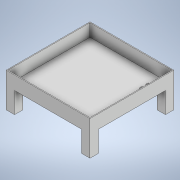
# Autodesk Inventor part: grow bed
Saved by Autodesk Inventor 2020 (Build 240168000, 168)
## iProperties
Created: 2019-09-26
Part Number: grow bed
Material: Generic
Document SubType Name: Modeling
Designer: Abbas
Density: 1 g/cm^3
Appearance: Default
Author: Abbas
Autodesk Inventor part; units mm, degrees
ref_plane "YZ Plane" through (0, 0, 0) normal (1, 0, 0) x (0, 1, 0)
ref_plane "XZ Plane" through (0, 0, 0) normal (0, 1, 0) x (-1, 0, 0)
ref_plane "XY Plane" through (0, 0, 0) normal (0, 0, 1) x (1, 0, 0)
sketch "Sketch2" plane through (0, 0, 0) normal (0, 1, 0) x (-1, 0, 0)
  line L0 (7.9621, 7.1123) -> (-1992.0379, 7.1123)
  line L1 (-1992.0379, 7.1123) -> (-1992.0379, -1992.8877)
  line L2 (-1992.0379, -1992.8877) -> (7.9621, -1992.8877)
  line L3 (7.9621, -1992.8877) -> (7.9621, 7.1123)
  point P0 (0, 0)
  dimension "d0" = 2000
  dimension "d1" = 2000
  constraints: 8 end point, 2 parallel, 1 horizontal, 1 perpendicular
  measures "d0" distance of L2.end L1.end
  measures "d1" distance of L1.end L0.end
extrude "Extrusion1" add sketch "Sketch2" along normal blind 320
sketch "Sketch5" plane through (0, 320, 0) normal (0, 1, 0) x (1, 0, 0)
  line L0 (12.0379, 12.8877) -> (1972.0379, 12.8877)
  line L1 (1972.0379, 12.8877) -> (1972.0379, 1972.8877)
  line L2 (1972.0379, 1972.8877) -> (12.0379, 1972.8877)
  line L3 (12.0379, 1972.8877) -> (12.0379, 12.8877)
  line L4 (-7.9621, -7.1123) -> (1992.0379, -7.1123) projected
  line L5 (1992.0379, -7.1123) -> (1992.0379, 1992.8877) projected
  dimension "d7" = 1960
  dimension "d8" = 20
  dimension "d9" = 1960
  dimension "d10" = 20
  constraints: 8 end point, 2 parallel, 1 horizontal, 1 perpendicular
  measures "d7" distance of L0.end L1.end
  measures "d8" distance between parallel lines of L4 L0
  measures "d9" distance of L1.end L2.end
  measures "d10" distance between parallel lines of L5 L1
extrude "Extrusion2" cut sketch "Sketch5" against normal blind 300
sketch "Sketch6" plane through (0, 20, 0) normal (0, 1, 0) x (1, 0, 0)
  circle A0 centre (1692.0379, 1692.8877) radius 50
  circle A1 centre (1692.0379, 1542.8877) radius 50
  line L0 (1992.0379, 1992.8877) -> (-7.9621, 1992.8877) projected
  line L1 (1992.0379, -7.1123) -> (1992.0379, 1992.8877) projected
  point P0 (0, 0)
  dimension "d13" = 100
  dimension "d14" = 100
  dimension "d15" = 300
  dimension "d16" = 300
  dimension "d17" = 300
  dimension "d18" = 150
  constraints: 2 centre point
  measures "d13" diameter of A1
  measures "d14" diameter of A0
  measures "d15" distance from line of L0 A0.centre
  measures "d16" distance from line of L1 A0.centre
  measures "d17" distance from line of L1 A1.centre
  measures "d18" distance of A1.centre A0.centre
extrude "Extrusion3" cut sketch "Sketch6" against normal blind 300
sketch "Sketch7" plane through (0, 0, 0) normal (0, -1, 0) x (1, 0, 0)
  line L0 (1992.0379, 7.1123) -> (1792.0379, 7.1123)
  line L1 (1792.0379, 7.1123) -> (1792.0379, -192.8877)
  line L2 (1792.0379, -192.8877) -> (1992.0379, -192.8877)
  line L3 (1992.0379, -192.8877) -> (1992.0379, 7.1123)
  line L4 (-7.9621, 7.1123) -> (1992.0379, 7.1123) projected
  line L5 (-7.9621, 7.1123) -> (192.0379, 7.1123)
  line L6 (192.0379, 7.1123) -> (192.0379, -192.8877)
  line L7 (192.0379, -192.8877) -> (-7.9621, -192.8877)
  line L8 (-7.9621, -192.8877) -> (-7.9621, 7.1123)
  line L9 (1792.0379, -1992.8877) -> (1792.0379, -1792.8877)
  line L10 (1792.0379, -1792.8877) -> (1992.0379, -1792.8877)
  line L11 (1992.0379, -1792.8877) -> (1992.0379, -1992.8877)
  line L12 (-7.9621, -1992.8877) -> (192.0379, -1992.8877)
  line L13 (192.0379, -1992.8877) -> (192.0379, -1792.8877)
  line L14 (192.0379, -1792.8877) -> (-7.9621, -1792.8877)
  line L15 (-7.9621, -1792.8877) -> (-7.9621, -1992.8877)
  point P0 (0, 0)
  point P1 (0, -1985.7753)
  dimension "d23" = 200
  dimension "d24" = 200
  constraints: 30 end point, 2 parallel, 1 horizontal, 1 perpendicular
  measures "d23" distance of L0.end L1.end
  measures "d24" distance of L1.end L2.end
extrude "Extrusion4" add sketch "Sketch7" along normal blind 500
sketch "Sketch8" plane through (0, 0, 0) normal (0, -1, 0) x (1, 0, 0)
  line L0 (1992.0379, -1992.8877) -> (-7.9621, -1992.8877) projected
  line L1 (1992.0379, -1992.8877) -> (1792.0379, -1992.8877)
  line L2 (1792.0379, -1992.8877) -> (1792.0379, -1792.8877)
  line L3 (1792.0379, -1792.8877) -> (1992.0379, -1792.8877)
  line L4 (1992.0379, -1792.8877) -> (1992.0379, -1992.8877)
  point P0 (0, 0)
  dimension "d27" = 200
  dimension "d28" = 200
  constraints: 8 end point, 2 parallel, 1 horizontal, 1 perpendicular
  measures "d27" distance of L2.end L3.end
  measures "d28" distance of L1.end L2.end
extrude "Extrusion5" add sketch "Sketch8" along normal blind 500
body "Solid1"
